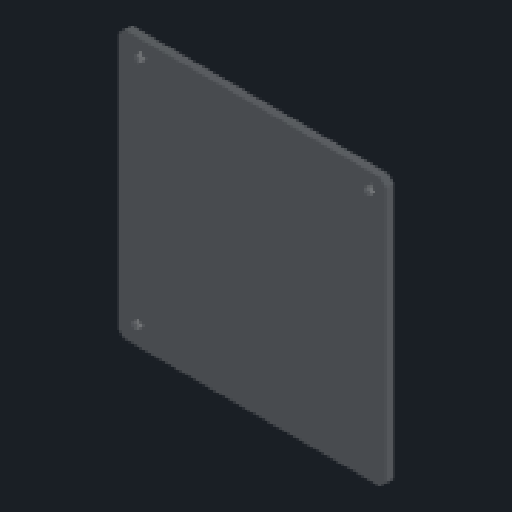
# Autodesk Inventor part: Buttom_acrylic
Saved by Autodesk Inventor 2026.2 (Build 302298000, 298)
## iProperties
Created: 2026-04-26
Part Number: Buttom_acrylic
Material: Generic
Document SubType Name: Modeling
Designer: Malthe Sennels
Density: 1 g/cm^3
Appearance: Polycarbonate - Clear
Author: Malthe Sennels
Autodesk Inventor part; units mm, degrees
ref_plane "YZ Plane" through (0, 0, 0) normal (1, 0, 0) x (0, 1, 0)
ref_plane "XZ Plane" through (0, 0, 0) normal (0, 1, 0) x (-1, 0, 0)
ref_plane "XY Plane" through (0, 0, 0) normal (0, 0, 1) x (1, 0, 0)
sketch "Sketch1" plane through (0, 0, 0) normal (0, 0, 1) x (1, 0, 0)
  line L0 (-49.9941, 52.4) -> (-52.4, 49.9941) projected
  line L1 (49.9941, 52.4) -> (-49.9941, 52.4) projected
  line L2 (52.4, 49.9941) -> (49.9941, 52.4) projected
  line L3 (49.9941, -52.4) -> (52.4, -49.9941) projected
  line L4 (-49.9941, -52.4) -> (49.9941, -52.4) projected
  line L5 (-52.4, -49.9941) -> (-49.9941, -52.4) projected
  line L6 (-52.4, -49.9941) -> (-52.4, 49.9941)
  line L7 (52.4, 49.9941) -> (52.4, -49.9941)
  circle A0 centre (-45.9242, -45.9242) radius 1.25 projected
  circle A1 centre (-44.8952, 45.0207) radius 1.25 projected
  circle A2 centre (45, 45) radius 1.25 projected
  point P0 (0, 0)
  constraints: 4 end point, 1 parallel, 1 vertical
extrude "Extrusion1" add sketch "Sketch1" along normal blind 3
body "Solid1"
